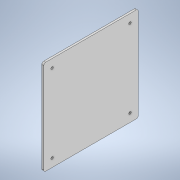
# Autodesk Inventor part: Plate
Saved by Autodesk Inventor 2022 (Build 260153000, 153)
## iProperties
Created: 2022-03-14
Part Number: Plate
Material: Generic
Document SubType Name: Modeling
Designer: ultra
Density: 1 g/cm^3
Appearance: Default
Author: ultra
Autodesk Inventor part; units mm, degrees
ref_plane "YZ Plane" through (0, 0, 0) normal (1, 0, 0) x (0, 1, 0)
ref_plane "XZ Plane" through (0, 0, 0) normal (0, 1, 0) x (-1, 0, 0)
ref_plane "XY Plane" through (0, 0, 0) normal (0, 0, 1) x (1, 0, 0)
sketch "Sketch1" plane through (0, 0, 0) normal (1, 0, 0) x (0, 1, 0)
  line L0 (-76.2, 76.2) -> (76.2, 76.2)
  line L1 (76.2, 76.2) -> (76.2, -76.2)
  line L2 (76.2, -76.2) -> (-76.2, -76.2)
  line L3 (-76.2, -76.2) -> (-76.2, 76.2)
  circle A0 centre (62.8611, 62.86) radius 2.032
  circle A1 centre (-62.8625, -62.8636) radius 2.032
  circle A2 centre (-0.0007, -88.9018) radius 2.032
  circle A3 centre (-62.8625, 62.86) radius 2.032
  circle A4 centre (88.8993, -0.0018) radius 2.032
  circle A5 centre (-88.9007, -0.0018) radius 2.032
  circle A6 centre (62.8611, -62.8636) radius 2.032
  circle A7 centre (-0.0007, 88.8982) radius 2.032
  circle A8 centre (-0.0007, -0.0018) radius 6.35
  dimension "d0" = 152.4
  dimension "d1" = 152.4
  dimension "d5" = 12.7
  constraints: 9 centre point, 8 end point, 2 parallel, 1 horizontal, 1 perpendicular
  measures "d0" distance of L1.end L2.end
  measures "d1" distance of L0.end L1.end
  measures "d5" diameter of A8
extrude "Extrusion2" add sketch "Sketch1" along normal blind 3.175 contours L0 L1 L2 L3 | A8
fillet "Fillet2" radius 3.175 4 edges at (1.5875, 76.2, 76.2) (1.5875, 76.2, -76.2) (1.5875, -76.2, 76.2) (1.5875, -76.2, -76.2)
body "Solid2"
